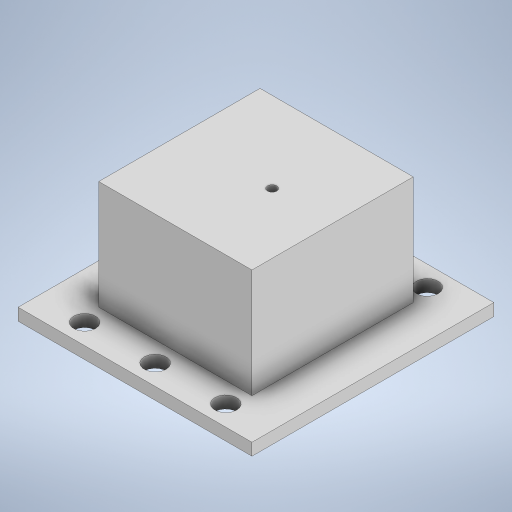
# Autodesk Inventor part: liquid_port_v06
Saved by Autodesk Inventor 2024 (Build 280153000, 153)
## iProperties
Created: 2021-04-13
Part Number: liquid_port_v06
Material: Generic
Document SubType Name: Modeling
Designer: KAMPFF-LAB-BEHAVIOR
Density: 1 g/cm^3
Appearance: Default
Author: KAMPFF-LAB-BEHAVIOR
Autodesk Inventor part; units mm, degrees
ref_plane "YZ Plane" through (0, 0, 0) normal (1, 0, 0) x (0, 1, 0)
ref_plane "XZ Plane" through (0, 0, 0) normal (0, 1, 0) x (-1, 0, 0)
ref_plane "XY Plane" through (0, 0, 0) normal (0, 0, 1) x (1, 0, 0)
ref_plane "Work Plane5" through (0, 3, 0) normal (0, 1, 0) x (1, 0, 0)
sketch "Sketch45" plane through (0, 3, 0) normal (0, 1, 0) x (1, 0, 0)
  line L0 (35, -20) -> (-3, -20)
  line L1 (-3, -20) -> (-3, 20)
  line L2 (-3, 20) -> (35, 20)
  line L3 (35, 20) -> (35, -20)
  point P0 (0, 0)
  dimension "d142" = 38
  dimension "d143" = 40
  constraints: 8 end point, 2 parallel, 1 horizontal, 1 perpendicular
  measures "d142" distance of L1.end L2.end
  measures "d143" distance of L0.end L1.end
extrude "Extrusion34" add sketch "Sketch45" along normal blind 30
ref_plane "Work Plane2" through (0, 0, 0) normal (0, -1, 0) x (1, 0, 0)
sketch "Sketch47" plane through (0, 0, 0) normal (0, -1, 0) x (1, 0, 0)
  circle A0 centre (16, 0) radius 18
  point P0 (0, 0)
  dimension "d146" = 36
  constraints: 1 centre point
  measures "d146" diameter of A0
extrude "Extrusion35" cut sketch "Sketch47" against normal blind 30 draft -15
ref_plane "Work Plane1" through (0, 3, 0) normal (0, 1, 0) x (1, 0, 0)
sketch "Sketch74" plane through (0, 33, 0) normal (0, 1, 0) x (1, 0, 0)
  circle A0 centre (20, 0) radius 1.15
  point P0 (0, 0)
  dimension "d210" = 2.3
  constraints: 1 centre point
  measures "d210" diameter of A0
extrude "Extrusion51" cut sketch "Sketch74" against normal blind 10
sketch "Sketch77" plane through (0, 3, 0) normal (0, -1, 0) x (1, 0, 0)
  circle A0 centre (16, 0) radius 17.5
  point P0 (0, 0)
  dimension "d219" = 35
  constraints: 1 centre point
  measures "d219" diameter of A0
sketch "Sketch78" plane through (0, 3, 0) normal (0, -1, 0) x (1, 0, 0)
  line L0 (45, -30) -> (-13, -30)
  line L1 (-13, -30) -> (-13, 30)
  line L2 (-13, 30) -> (45, 30)
  line L3 (45, 30) -> (45, -30)
  line L4 (45, -30) -> (-13, 30) construction
  line L5 (-13, -30) -> (45, 30) construction
  point P0 (0, 0)
  point P1 (16, 0)
  dimension "d220" = 58
  dimension "d221" = 60
  constraints: 12 end point, 2 midpoint, 2 parallel, 1 horizontal, 1 perpendicular
  measures "d220" distance of L1.end L2.end
  measures "d221" distance of L0.end L1.end
extrude "Extrusion53" add sketch "Sketch78" against normal blind 3
extrude "Extrusion54" cut sketch "Sketch77" against normal blind 3
sketch "Sketch81" plane through (0, 3, 0) normal (0, -1, 0) x (1, 0, 0)
  circle A0 centre (33.5, -25) radius 2.7
  line L0 (-13, -30) -> (45, -30) projected
  line L1 (45, -30) -> (45, 30) projected
  circle A1 centre (16, -25) radius 2.7
  circle A2 centre (-1.5, -25) radius 2.7
  circle A3 centre (-1.5, 25) radius 2.7
  circle A4 centre (16, 25) radius 2.7
  circle A5 centre (33.5, 25) radius 2.7
  point P0 (0, 0)
  dimension "mag_D" = 5.4
  dimension "d232" = 5
  dimension "d233" = 11.5
  dimension "d234" = 5.4
  dimension "d235" = 17.5
  dimension "d236" = 5.4
  dimension "d237" = 17.5
  dimension "d243" = 5.4
  dimension "d245" = 5.4
  dimension "d246" = 17.5
  dimension "d247" = 5.4
  dimension "d248" = 17.5
  constraints: 6 centre point
  measures "mag_D" diameter of A0
  measures "d232" distance from line of A0.centre L0
  measures "d233" distance from line of L1 A0.centre
  measures "d234" diameter of A1
  measures "d235" distance of A0.centre A1.centre
  measures "d236" diameter of A2
  measures "d237" distance of A1.centre A2.centre
  measures "d243" diameter of A3
  measures "d245" diameter of A4
  measures "d246" distance of A4.centre A3.centre
  measures "d247" diameter of A5
  measures "d248" distance of A5.centre A4.centre
extrude "Extrusion56" cut sketch "Sketch81" against normal blind 30
equation "\"d234\" = mag_D"
equation "\"d236\" = mag_D"
equation "\"d237\" = d235"
equation "\"d243\" = mag_D"
equation "\"d245\" = mag_D"
equation "\"d246\" = d235"
equation "\"d247\" = mag_D"
equation "\"d248\" = d235"
body "Solid9"
